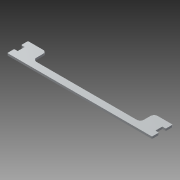
# Autodesk Inventor part: Bulkhead Brace 25100613
Saved by Autodesk Inventor 2013 (Build 170138000, 138)
## iProperties
Created: 2012-05-10
Part Number: Bulkhead Brace 25100613
Material: Generic
Document SubType Name: Modeling
Designer: user
Density: 1 g/cm^3
Author: user
Autodesk Inventor part; units mm, degrees
ref_plane "YZ Plane" through (0, 0, 0) normal (1, 0, 0) x (0, 1, 0)
ref_plane "XZ Plane" through (0, 0, 0) normal (0, 1, 0) x (-1, 0, 0)
ref_plane "XY Plane" through (0, 0, 0) normal (0, 0, 1) x (1, 0, 0)
sketch "Sketch1" plane through (0, 0, 0) normal (0, 0, 1) x (1, 0, 0)
  line L0 (1, 0) -> (209, 0)
  line L1 (178, 10) -> (32, 10)
  arc A0 (209, 0) -> (210, 1) centre (209, 1) ccw
  arc A1 (0, 1) -> (1, 0) centre (1, 1) ccw
  line L2 (27, 15) -> (27, 25)
  line L3 (22, 30) -> (1, 30)
  line L4 (1, 10) -> (5, 10)
  line L5 (5, 10) -> (5, 20)
  line L6 (5, 20) -> (1, 20)
  line L7 (0, 29) -> (0, 21)
  line L8 (0, 9) -> (0, 1)
  arc A2 (1, 30) -> (0, 29) centre (1, 29) ccw
  arc A3 (0, 21) -> (1, 20) centre (1, 21) ccw
  arc A4 (1, 10) -> (0, 9) centre (1, 9) ccw
  line L9 (183, 15) -> (183, 25)
  line L10 (188, 30) -> (209, 30)
  line L11 (209, 20) -> (205, 20)
  line L12 (205, 20) -> (205, 10)
  line L13 (205, 10) -> (209, 10)
  line L14 (210, 1) -> (210, 9)
  line L15 (210, 21) -> (210, 29)
  arc A5 (210, 29) -> (209, 30) centre (209, 29) ccw
  arc A6 (209, 20) -> (210, 21) centre (209, 21) ccw
  arc A7 (210, 9) -> (209, 10) centre (209, 9) ccw
  arc A8 (27, 25) -> (22, 30) centre (22, 25) ccw
  arc A9 (27, 15) -> (32, 10) centre (32, 15) ccw
  arc A10 (178, 10) -> (183, 15) centre (178, 15) ccw
  arc A11 (188, 30) -> (183, 25) centre (188, 25) ccw
  point P0 (0, 0)
  point P1 (183, 10)
  point P2 (27, 10)
  point P3 (27, 30)
  point P4 (0, 30)
  point P5 (210, 30)
  point P6 (183, 30)
  point P7 (210, 20)
  point P8 (210, 10)
  dimension "d0" = 10
  dimension "d2" = 1
  dimension "d8" = 27
  dimension "d9" = 10
  dimension "d11" = 5
  dimension "d12" = 1
  dimension "d13" = 27
  dimension "d14" = 5
  dimension "d15" = 10
  dimension "d16" = 10
  dimension "d17" = 30
  dimension "d18" = 1
  dimension "d19" = 30
  dimension "d20" = 210
  dimension "d21" = 5
  constraints: 32 end point, 26 tangent, 24 point on circle, 17 point on line, 12 centre point, 10 parallel, 10 perpendicular, 7 equal radius, 1 horizontal
  measures "d0" distance between parallel lines of L0 L1
  measures "d2" radius of A0
  measures "d8" distance of point (27, 30) point (0, 30)
  measures "d9" distance between parallel lines of L6 L3
  measures "d11" distance between parallel lines of L5 L7
  measures "d12" radius of A2
  measures "d13" distance of point (183, 30) point (210, 30)
  measures "d14" distance of point (210, 20) L11.end
  measures "d15" distance of point (210, 20) point (210, 30)
  measures "d16" distance between parallel lines of L0 L13
  measures "d17" distance between parallel lines of L0 L10
  measures "d18" radius of A5
  measures "d19" distance between parallel lines of L0 L3
  measures "d20" distance between parallel lines of L14 L8
  measures "d21" radius of A8
extrude "Extrusion1" add sketch "Sketch1" along normal blind 3
body "Solid1"
